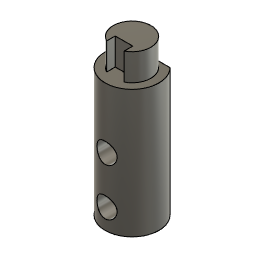
toolholder_torgs v2 (Autodesk Fusion 360 design; units mm, degrees)
Autodesk Fusion 360 part; units mm, degrees
sketch "Sketch1" plane through (0, 0, 0) normal (0, 1, 0) x (1, 0, 0)
  circle A0 centre (0, 0) radius 2.8
  circle A1 centre (0, 0) radius 4
  line L0 (0, 2.8) -> (2.8566, 2.8)
  line L1 (0, 2.8) -> (-2.8566, 2.8)
  line L2 (0, 0) -> (0, -1.2)
  line L3 (0, -1.2) -> (1.3, -1.2)
  line L4 (0, -1.2) -> (-1.3, -1.2)
  line L5 (-1.3, -1.2) -> (-1.3, -2.4799)
  line L6 (1.3, -1.2) -> (1.3, -2.4799)
  dimension "d1" = 5.6
  dimension "d2" = 8
  dimension "d22" = 1.2
  dimension "d23" = 1.3
  dimension "d24" = 1.3
  constraint coincident A0.centre A1.centre
  constraint coincident A0 L0.start
  constraint coincident A1 L0.end
  constraint tangent A0 L0
  constraint coincident A1 L1.end
  constraint tangent A0 L1
  constraint perpendicular L2 L3
  constraint perpendicular L2 L4
  constraint coincident A0 L5.end
  constraint perpendicular L4 L5
  constraint coincident A0 L6.end
  constraint perpendicular L3 L6
  measures "d1" diameter of A0
  measures "d2" diameter of A1
  measures "d22" distance of A0.centre L2.end
  measures "d23" distance of L2.end L3.end
  measures "d24" distance of L2.end L4.end
extrude "Extrude1" add sketch "Sketch1" along normal blind 6 contours A0 L3 L4 L5 L6 picked at (1.1387, -0.1888)
extrude "Extrude2" add sketch "Sketch1" along normal blind 2 contours A0 L3 L4 L5 L6 | A1 L0 L1 | A0 L3 L4 L5 L6 picked at (1.668, -3.1824)
extrude "Extrude3" add sketch "Sketch1" against normal blind 17 contours A0 L3 L4 L5 L6 | A1 L0 L1 | A0 L3 L4 L5 L6 picked at (1.668, -3.1824)
sketch "Sketch2" plane through (0, 0, -2.8) normal (0, 0, -1) x (-1, 0, 0)
  line L0 (-2.8566, 2) -> (-2.8566, -17)
  line L1 (0, 2) -> (-2.8566, 2)
  line L2 (-2.8566, -17) -> (2.8566, -17)
  line L3 (0, 0) -> (0, -14)
  circle A0 centre (0, -14) radius 1.5
  line L4 (2.8566, -17) -> (2.8566, 2)
  line L5 (2.8566, 2) -> (0, 2)
  circle A1 centre (0, -7) radius 1.5
  dimension "d13" = 14
  dimension "d14" = 3
  dimension "d25" = 3
  constraint coincident L3.start origin
  constraint coincident L3.end A0.centre
  constraint midpoint L3 A1.centre
  measures "d13" distance of L3.start L3.end
  measures "d14" diameter of A0
  measures "d25" diameter of A1
extrude "Extrude4" cut sketch "Sketch2" against normal blind 7 contours L3 A1 | L3 A1 | A0
